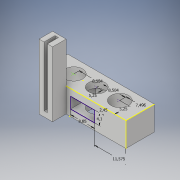
# Autodesk Inventor part: Objektträgerhalter 2bfinal
Saved by Autodesk Inventor 2018.3 (Build 223284000, 284)
## iProperties
Created: 2018-12-06
Part Number: Objektträgerhalter 2bfinal
Material: Generisch
Document SubType Name: Modeling
Designer: pgmadmin
Density: 1 g/cm^3
Appearance: Vorgabe
Author: pgmadmin
Autodesk Inventor part; units mm, degrees
ref_plane "YZ Plane" through (0, 0, 0) normal (1, 0, 0) x (0, 1, 0)
ref_plane "XZ Plane" through (0, 0, 0) normal (0, 1, 0) x (-1, 0, 0)
ref_plane "XY Plane" through (0, 0, 0) normal (0, 0, 1) x (1, 0, 0)
sketch "Skizze1" plane through (0, 0, 0) normal (0, 0, 1) x (1, 0, 0)
  line L0 (-11.356, -4.7452) -> (20.644, -4.7452)
  line L1 (20.644, -4.7452) -> (20.644, 5.7548)
  line L2 (20.644, 5.7548) -> (-11.356, 5.7548)
  line L3 (-11.356, 5.7548) -> (-11.356, -4.7452)
  point P0 (0, 0)
  dimension "d0" = 32
  dimension "d1" = 10.5
  constraints: 8 end point, 2 parallel, 1 horizontal, 1 perpendicular
  measures "d0" distance of L2.end L1.end
  measures "d1" distance of L1.end L0.end
extrude "Extrusion1" add sketch "Skizze1" along normal blind 9
sketch "Skizze2" plane through (0, 0, 9) normal (0, 0, 1) x (1, 0, 0)
  line L0 (20.644, -4.7452) -> (20.644, 5.7548) projected
  line L1 (-11.356, -4.7452) -> (20.644, -4.7452) projected
  point P0 (0, 0)
  point P1 (-3.86, 0.5048)
  point P2 (4.644, 0.5048)
  point P3 (13.148, 0.5048)
  dimension "d4" = 8.504
  dimension "d5" = 8.504
  dimension "d6" = 7.496
  dimension "d20" = 5.25
  dimension "d21" = 5.25
  measures "d4" distance of point (4.644, 0.505) point (-3.86, 0.505)
  measures "d5" distance of point (4.644, 0.505) point (13.148, 0.505)
  measures "d6" distance from line of L0 point (13.148, 0.505)
  measures "d20" distance from line of L1 point (4.644, 0.505)
  measures "d21" distance from line of L1 point (13.148, 0.505)
sketch "Skizze3" plane through (0, 0, 9) normal (0, 0, 1) x (1, 0, 0)
  point P0 (0, 0)
sketch "Skizze4" plane through (-11.356, -4.7452, 0) normal (0, -1, 0) x (1, 0, 0)
  line L0 (11.575, 6.55) -> (20.425, 6.55)
  line L1 (20.425, 6.55) -> (20.425, 2.45)
  line L2 (20.425, 2.45) -> (11.575, 2.45)
  line L3 (11.575, 2.45) -> (11.575, 6.55)
  line L4 (32, 0) -> (32, 9) projected
  line L5 (0, 9) -> (32, 9) projected
  point P0 (11.356, 0)
  dimension "d14" = 8.85
  dimension "d15" = 4.1
  dimension "d16" = 11.575
  dimension "d17" = 2.45
  constraints: 8 end point, 2 parallel, 1 horizontal, 1 perpendicular
  measures "d14" distance of L1.end L2.end
  measures "d15" distance of L0.end L1.end
  measures "d16" distance between parallel lines of L4 L1
  measures "d17" distance between parallel lines of L5 L0
extrude "Extrusion2" cut sketch "Skizze4" against normal blind 9.3
sketch "Skizze5" plane through (0, 0, 9) normal (0, 0, 1) x (1, 0, 0)
  point P0 (0, 0)
sketch "Skizze6" plane through (-11.356, -4.7452, 0) normal (0, -1, 0) x (1, 0, 0)
  line L0 (4.905, 0) -> (9.905, 0)
  line L1 (9.905, 0) -> (9.905, 2)
  line L2 (9.905, 2) -> (4.905, 2)
  line L3 (4.905, 2) -> (4.905, 0)
  line L4 (0, 0) -> (0, 9) projected
  point P0 (11.356, 0)
  dimension "d22" = 5
  dimension "d23" = 2
  dimension "d24" = 4.905
  constraints: 8 end point, 2 parallel, 1 horizontal, 1 perpendicular
  measures "d22" distance of L2.end L1.end
  measures "d23" distance between parallel lines of L0 L2
  measures "d24" distance between parallel lines of L3 L4
sketch "Skizze7" plane through (-11.356, -4.7452, 0) normal (0, -1, 0) x (1, 0, 0)
  point P0 (11.356, 0)
extrude "Extrusion3" add sketch "Skizze6" along normal blind 5
sketch "Skizze8" plane through (-6.451, -4.7452, 2) normal (0, 0, 1) x (1, 0, 0)
  line L0 (0, -5) -> (5, -5) projected
  line L1 (0, 0) -> (0, -5) projected
  line L2 (5, -5) -> (0, -5)
  line L3 (0, -5) -> (0, 0)
  line L4 (0, 0) -> (5, 0)
  line L5 (5, 0) -> (5, -5)
  point P0 (6.451, 4.7452)
  constraints: 8 end point, 2 parallel, 1 horizontal, 1 perpendicular
extrude "Extrusion4" add sketch "Skizze8" along normal blind 22
sketch "Skizze9" plane through (-6.451, -4.7452, 24) normal (0, 0, 1) x (1, 0, 0)
  line L0 (0, -5) -> (5, -5) projected
  line L1 (1.875, -5) -> (3.125, -5)
  line L2 (3.125, -5) -> (3.125, -0.952)
  line L3 (3.125, -0.952) -> (1.875, -0.952)
  line L4 (1.875, -0.952) -> (1.875, -5)
  line L5 (5, -5) -> (5, 0) projected
  line L6 (0, 0) -> (0, -5) projected
  point P0 (6.451, 4.7452)
  dimension "d29" = 1.875
  dimension "d30" = 1.875
  dimension "d31" = 4.048
  constraints: 8 end point, 2 parallel, 1 horizontal, 1 perpendicular, 1 point on line
  measures "d29" distance between parallel lines of L5 L2
  measures "d30" distance between parallel lines of L6 L4
  measures "d31" distance between parallel lines of L3 L0
extrude "Extrusion5" cut sketch "Skizze9" against normal blind 22
hole "Bohrung2" at (4.644, 0.5048, 9) direction (0, 0, -1) diameter 6 end through all
hole "Bohrung3" at (13.148, 0.5048, 9) at (-3.86, 0.5048, 9) direction (0, 0, -1) diameter 6.5 end through all
